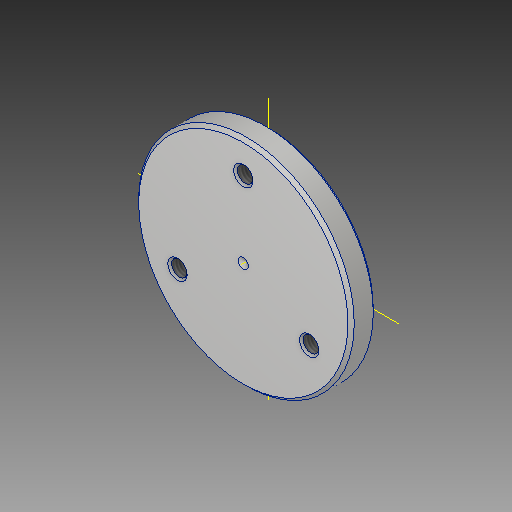
# Autodesk Inventor part: podporka_pajaka
Saved by Autodesk Inventor 2019.4 (Build 234330000, 330)
## iProperties
Created: 2019-05-25
Part Number: podporka_pajaka
Material: Aluminium 6061
Document SubType Name: Modeling
Designer: Esterka
Density: 2.7 g/cm^3
Appearance: Aluminium — płaski
Author: Esterka
Autodesk Inventor part; units mm, degrees
ref_plane "YZ Plane" through (0, 0, 0) normal (1, 0, 0) x (0, 1, 0)
ref_plane "XZ Plane" through (0, 0, 0) normal (0, 1, 0) x (-1, 0, 0)
sketch "Sketch1" plane through (0, 0, 0) normal (0, 0, 1) x (1, 0, 0)
  circle A0 centre (0, 0) radius 17
  dimension "d0" = 34
  constraints: 1 centre point, 1 coincident
  measures "d0" diameter of A0
extrude "Extrusion1" add sketch "Sketch1" along normal blind 4
sketch "Sketch2" plane through (0, 0, 0) normal (1, 0, 0) x (0, 1, 0)
  line L0 (17, 4) -> (-17, 4) projected
  line L1 (0, 4) -> (0.8, 4)
  line L2 (0, 4) -> (0, 3.5381)
  line L3 (0, 3.5381) -> (0.8, 4)
  line L4 (0, -0.8) -> (0, 4.8) projected
  point P0 (0, 0)
  dimension "d3" = 0.8
  dimension "d40" = 60
  constraints: 6 end point, 1 midpoint, 1 point on line, 1 vertical
  measures "d3" distance of L1.start L1.end
  measures "d40" angle of L3 L2
revolve "Revolution1" cut sketch "Sketch2" angle 360 about axis through (0, 0, -10) along (0, 0, 1)
ref_plane "Work Plane1" through (0, 0, 4) normal (0, 0, 1) x (1, 0, 0)
sketch "Sketch3" plane through (0, 0, 4) normal (0, 0, 1) x (1, 0, 0)
  circle A0 centre (0, 0) radius 12
  point P0 (0, 12)
  point P1 (-10.3923, -6)
  point P2 (10.3923, -6)
  dimension "d7" = 24
  dimension "d10" = 360
  constraints: 1 coincident, 1 vertical alignment, 6 other
hole "Hole7" at (0, 12, 4) at (-10.3923, -6, 4) at (10.3923, -6, 4) direction (0, 0, -1) diameter 2.459 end through all thread size "M3x0.5" class "6H" standard "ISO Metric profile"
chamfer "Chamfer2" distance 0.3 angle 45 3 edges at (-10.3923, -4.7705, 4) (10.3923, -4.7705, 4) (0, 13.2295, 4)
chamfer "Chamfer3" distance 0.5 angle 45 2 edges at (-17, 0, 4) (-17, 0, 0)
sketch "Sketch4" plane through (0, 0, 4) normal (0, 0, 1) x (1, 0, 0)
  point P0 (-51.4403, -28.5545)
  point P1 (-61.8326, -46.5545)
  point P2 (-72.2249, -28.5545)
sketch "Sketch5" plane through (0, 0, 4) normal (0, 0, 1) x (1, 0, 0)
  point P0 (-51.4403, -28.5545)
  point P1 (-61.8326, -46.5545)
  point P2 (-72.2249, -28.5545)
sketch "Sketch6" plane through (0, 0, 4) normal (0, 0, 1) x (1, 0, 0)
  point P0 (-51.4403, -28.5545)
body "Solid1"
